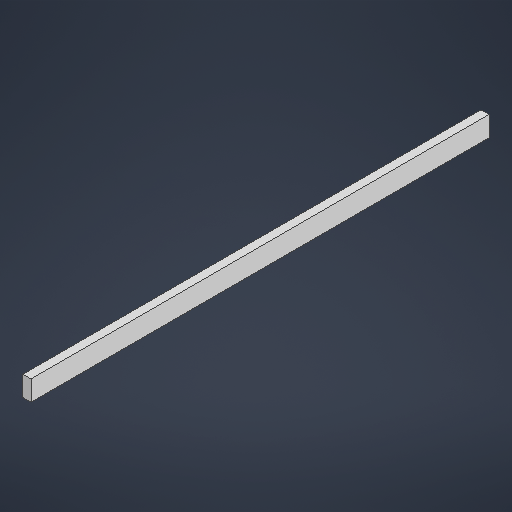
# Autodesk Inventor part: backwall
Saved by Autodesk Inventor 2026.2 (Build 302298010, 298A)
## iProperties
Created: 2026-03-30
Part Number: backwall
Material: Generic
Document SubType Name: Modeling
Designer: karol
Density: 1 g/cm^3
Appearance: Default
Author: karol
Autodesk Inventor part; units mm, degrees
ref_plane "YZ Plane" through (0, 0, 0) normal (1, 0, 0) x (0, 1, 0)
ref_plane "XZ Plane" through (0, 0, 0) normal (0, 1, 0) x (-1, 0, 0)
ref_plane "XY Plane" through (0, 0, 0) normal (0, 0, 1) x (1, 0, 0)
derived "base.ipt"
sketch "Sketch3" plane through (0, 0, 0) normal (0, 1, 0) x (-1, 0, 0)
  line L0 (0, 0) -> (170, 0) projected
  line L1 (170, 0) -> (170, -170) projected
  line L2 (170, -170) -> (0, -170) projected
  line L3 (0, -170) -> (0, 0) projected
  line L4 (170, 0) -> (167, 0) projected
  line L5 (167, 0) -> (167, -170) projected
  line L6 (167, -170) -> (170, -170) projected
  line L7 (170, -170) -> (170, 0) projected
  line L8 (167, 0) -> (148.6, 0) projected
  line L9 (148.6, 0) -> (148.6, -3) projected
  line L10 (148.6, -3) -> (167, -3) projected
  line L11 (167, -3) -> (167, 0) projected
  line L12 (148.6, -3) -> (151.6, -3) projected
  line L13 (151.6, -3) -> (151.6, -25) projected
  line L14 (151.6, -25) -> (148.6, -25) projected
  line L15 (148.6, -25) -> (148.6, -3) projected
  line L16 (167, -170) -> (148.6, -170) projected
  line L17 (148.6, -170) -> (148.6, -167) projected
  line L18 (148.6, -167) -> (167, -167) projected
  line L19 (167, -167) -> (167, -170) projected
  line L20 (148.6, -167) -> (151.6, -167) projected
  line L21 (151.6, -167) -> (151.6, -145) projected
  line L22 (151.6, -145) -> (148.6, -145) projected
  line L23 (148.6, -145) -> (148.6, -167) projected
  line L24 (167, -167) -> (152, -167) projected
  line L25 (152, -167) -> (152, -150.8) projected
  line L26 (152, -150.8) -> (167, -150.8) projected
  line L27 (167, -150.8) -> (167, -167) projected
  line L28 (167, -3) -> (152, -3) projected
  line L29 (152, -3) -> (152, -19.2) projected
  line L30 (152, -19.2) -> (167, -19.2) projected
  line L31 (167, -19.2) -> (167, -3) projected
  line L32 (148.6, -25) -> (118.6, -25) projected
  line L33 (118.6, -25) -> (118.6, 0) projected
  line L34 (118.6, 0) -> (148.6, 0) projected
  line L35 (148.6, 0) -> (148.6, -25) projected
  line L36 (148.6, -145) -> (118.6, -145) projected
  line L37 (118.6, -145) -> (118.6, -170) projected
  line L38 (118.6, -170) -> (148.6, -170) projected
  line L39 (148.6, -170) -> (148.6, -145) projected
  line L40 (0, 0) -> (20, 0) projected
  line L41 (20, 0) -> (20, -3) projected
  line L42 (20, -3) -> (0, -3) projected
  line L43 (0, -3) -> (0, 0) projected
  line L44 (0, -170) -> (20, -170) projected
  line L45 (20, -170) -> (20, -167) projected
  line L46 (20, -167) -> (0, -167) projected
  line L47 (0, -167) -> (0, -170) projected
  line L48 (20, -3) -> (5, -3) projected
  line L49 (5, -3) -> (5, -19.2) projected
  line L50 (5, -19.2) -> (20, -19.2) projected
  line L51 (20, -19.2) -> (20, -3) projected
  line L52 (20, -167) -> (5, -167) projected
  line L53 (5, -167) -> (5, -150.8) projected
  line L54 (5, -150.8) -> (20, -150.8) projected
  line L55 (20, -150.8) -> (20, -167) projected
  line L56 (20, 0) -> (23, 0) projected
  line L57 (23, 0) -> (23, -25) projected
  line L58 (23, -25) -> (20, -25) projected
  line L59 (20, -25) -> (20, 0) projected
  line L60 (23, -25) -> (53, -25) projected
  line L61 (53, -25) -> (53, 0) projected
  line L62 (53, 0) -> (23, 0) projected
  line L63 (23, 0) -> (23, -25) projected
  line L64 (53, 0) -> (56, 0) projected
  line L65 (56, 0) -> (56, -25) projected
  line L66 (56, -25) -> (53, -25) projected
  line L67 (53, -25) -> (53, 0) projected
  line L68 (53, -25) -> (23, -25) projected
  line L69 (23, -25) -> (23, -22) projected
  line L70 (23, -22) -> (53, -22) projected
  line L71 (53, -22) -> (53, -25) projected
  line L72 (148.6, -25) -> (118.6, -25) projected
  line L73 (118.6, -25) -> (118.6, -22) projected
  line L74 (118.6, -22) -> (148.6, -22) projected
  line L75 (148.6, -22) -> (148.6, -25) projected
  line L76 (118.6, -25) -> (115.6, -25) projected
  line L77 (115.6, -25) -> (115.6, 0) projected
  line L78 (115.6, 0) -> (118.6, 0) projected
  line L79 (118.6, 0) -> (118.6, -25) projected
  line L80 (148.6, -145) -> (118.6, -145) projected
  line L81 (118.6, -145) -> (118.6, -148) projected
  line L82 (118.6, -148) -> (148.6, -148) projected
  line L83 (148.6, -148) -> (148.6, -145) projected
  line L84 (118.6, -145) -> (115.6, -145) projected
  line L85 (115.6, -145) -> (115.6, -170) projected
  line L86 (115.6, -170) -> (118.6, -170) projected
  line L87 (118.6, -170) -> (118.6, -145) projected
  line L88 (20, -170) -> (23, -170) projected
  line L89 (23, -170) -> (23, -145) projected
  line L90 (23, -145) -> (20, -145) projected
  line L91 (20, -145) -> (20, -170) projected
  line L92 (23, -170) -> (53, -170) projected
  line L93 (53, -170) -> (53, -145) projected
  line L94 (53, -145) -> (23, -145) projected
  line L95 (23, -145) -> (23, -170) projected
  line L96 (53, -145) -> (56, -145) projected
  line L97 (56, -145) -> (56, -170) projected
  line L98 (56, -170) -> (53, -170) projected
  line L99 (53, -170) -> (53, -145) projected
  line L100 (53, -145) -> (23, -145) projected
  line L101 (23, -145) -> (23, -148) projected
  line L102 (23, -148) -> (53, -148) projected
  line L103 (53, -148) -> (53, -145) projected
  line L104 (148.6, -25) -> (146.6, -25) projected
  line L105 (146.6, -25) -> (146.6, -49) projected
  line L106 (146.6, -49) -> (148.6, -49) projected
  line L107 (148.6, -49) -> (148.6, -25) projected
  line L108 (118.6, -25) -> (120.6, -25) projected
  line L109 (120.6, -25) -> (120.6, -49) projected
  line L110 (120.6, -49) -> (118.6, -49) projected
  line L111 (118.6, -49) -> (118.6, -25) projected
  line L112 (146.6, -25) -> (134.6, -25) projected
  line L113 (134.6, -25) -> (134.6, -49) projected
  line L114 (134.6, -49) -> (146.6, -49) projected
  line L115 (146.6, -49) -> (146.6, -25) projected
  line L116 (120.6, -49) -> (132.6, -49) projected
  line L117 (132.6, -49) -> (132.6, -25) projected
  line L118 (132.6, -25) -> (120.6, -25) projected
  line L119 (120.6, -25) -> (120.6, -49) projected
  line L120 (148.6, -145) -> (146.6, -145) projected
  line L121 (146.6, -145) -> (146.6, -121) projected
  line L122 (146.6, -121) -> (148.6, -121) projected
  line L123 (148.6, -121) -> (148.6, -145) projected
  line L124 (118.6, -145) -> (120.6, -145) projected
  line L125 (120.6, -145) -> (120.6, -121) projected
  line L126 (120.6, -121) -> (118.6, -121) projected
  line L127 (118.6, -121) -> (118.6, -145) projected
  line L128 (146.6, -121) -> (134.6, -121) projected
  line L129 (134.6, -121) -> (134.6, -145) projected
  line L130 (134.6, -145) -> (146.6, -145) projected
  line L131 (146.6, -145) -> (146.6, -121) projected
  line L132 (120.6, -121) -> (132.6, -121) projected
  line L133 (132.6, -121) -> (132.6, -145) projected
  line L134 (132.6, -145) -> (120.6, -145) projected
  line L135 (120.6, -145) -> (120.6, -121) projected
  line L136 (53, -25) -> (51, -25) projected
  line L137 (51, -25) -> (51, -60.37) projected
  line L138 (51, -60.37) -> (53, -60.37) projected
  line L139 (53, -60.37) -> (53, -25) projected
  line L140 (51, -25) -> (39, -25) projected
  line L141 (39, -25) -> (39, -60.37) projected
  line L142 (39, -60.37) -> (51, -60.37) projected
  line L143 (51, -60.37) -> (51, -25) projected
  line L144 (23, -25) -> (25, -25) projected
  line L145 (25, -25) -> (25, -60.37) projected
  line L146 (25, -60.37) -> (23, -60.37) projected
  line L147 (23, -60.37) -> (23, -25) projected
  line L148 (25, -25) -> (37, -25) projected
  line L149 (37, -25) -> (37, -60.37) projected
  line L150 (37, -60.37) -> (25, -60.37) projected
  line L151 (25, -60.37) -> (25, -25) projected
  line L152 (53, -145) -> (51, -145) projected
  line L153 (51, -145) -> (51, -121) projected
  line L154 (51, -121) -> (53, -121) projected
  line L155 (53, -121) -> (53, -145) projected
  line L156 (51, -121) -> (39, -121) projected
  line L157 (39, -121) -> (39, -145) projected
  line L158 (39, -145) -> (51, -145) projected
  line L159 (51, -145) -> (51, -121) projected
  line L160 (23, -145) -> (25, -145) projected
  line L161 (25, -145) -> (25, -121) projected
  line L162 (25, -121) -> (23, -121) projected
  line L163 (23, -121) -> (23, -145) projected
  line L164 (25, -121) -> (37, -121) projected
  line L165 (37, -121) -> (37, -145) projected
  line L166 (37, -145) -> (25, -145) projected
  line L167 (25, -145) -> (25, -121) projected
  line L168 (118.6, -25) -> (115.6, -25) projected
  line L169 (115.6, -25) -> (115.6, 0) projected
  line L170 (115.6, 0) -> (118.6, 0) projected
  line L171 (118.6, 0) -> (118.6, -25) projected
  line L172 (115.6, 0) -> (56, 0) projected
  line L173 (56, 0) -> (56, -3) projected
  line L174 (56, -3) -> (115.6, -3) projected
  line L175 (115.6, -3) -> (115.6, 0) projected
  line L176 (115.6, -170) -> (56, -170) projected
  line L177 (56, -170) -> (56, -167) projected
  line L178 (56, -167) -> (115.6, -167) projected
  line L179 (115.6, -167) -> (115.6, -170) projected
  line L180 (51, -25) -> (39, -25) projected
  line L181 (39, -25) -> (39, -49) projected
  line L182 (39, -49) -> (51, -49) projected
  line L183 (51, -49) -> (51, -25) projected
  line L184 (37, -25) -> (25, -25) projected
  line L185 (25, -25) -> (25, -49) projected
  line L186 (25, -49) -> (37, -49) projected
  line L187 (37, -49) -> (37, -25) projected
extrude "Extrusion1" add sketch "Sketch3" along normal blind 7.5 contours L0 L1 L2 L5
body "Solid1"
